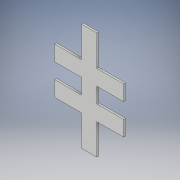
# Autodesk Inventor part: backplatelift
Saved by Autodesk Inventor 2017 (Build 210142000, 142)
## iProperties
Created: 2017-05-30
Part Number: backplatelift
Material: Generic
Document SubType Name: Modeling
Designer: User
Density: 1 g/cm^3
Appearance: Default
Author: User
Autodesk Inventor part; units mm, degrees
ref_plane "YZ Plane" through (0, 0, 0) normal (1, 0, 0) x (0, 1, 0)
ref_plane "XZ Plane" through (0, 0, 0) normal (0, 1, 0) x (-1, 0, 0)
ref_plane "XY Plane" through (0, 0, 0) normal (0, 0, 1) x (1, 0, 0)
sketch "Sketch1" plane through (0, 0, 0) normal (0, 0, 1) x (1, 0, 0)
  line L0 (0, 0) -> (50.8, 0)
  line L1 (50.8, 0) -> (50.8, 355.6)
  line L2 (50.8, 355.6) -> (0, 355.6)
  line L3 (0, 355.6) -> (0, 0)
  dimension "d0" = 50.8
  dimension "d1" = 355.6
  constraints: 8 end point, 2 parallel, 1 horizontal, 1 perpendicular
  measures "d0" distance of L2.end L1.end
  measures "d1" distance of L1.end L0.end
extrude "Extrusion1" add sketch "Sketch1" along normal blind 6.35
sketch "Sketch2" plane through (0, 0, 6.35) normal (0, 0, 1) x (1, 0, 0)
  line L0 (50.8, 0) -> (50.8, 355.6) projected
  line L1 (50.8, 152.4) -> (50.8, 203.2)
  line L2 (0, 152.4) -> (0, 203.2)
  line L3 (0, 355.6) -> (0, 0) projected
  line L4 (-88.9, 254) -> (0, 254)
  line L5 (0, 254) -> (0, 203.2)
  line L6 (0, 203.2) -> (-88.9, 203.2)
  line L7 (-88.9, 203.2) -> (-88.9, 254)
  line L8 (-88.9, 152.4) -> (0, 152.4)
  line L9 (0, 152.4) -> (0, 101.6)
  line L10 (0, 101.6) -> (-88.9, 101.6)
  line L11 (-88.9, 101.6) -> (-88.9, 152.4)
  line L12 (50.8, 101.6) -> (139.7, 101.6)
  line L13 (139.7, 101.6) -> (139.7, 152.4)
  line L14 (139.7, 152.4) -> (50.8, 152.4)
  line L15 (50.8, 152.4) -> (50.8, 101.6)
  line L16 (139.7, 203.2) -> (50.8, 203.2)
  line L17 (50.8, 203.2) -> (50.8, 254)
  line L18 (50.8, 254) -> (139.7, 254)
  line L19 (139.7, 254) -> (139.7, 203.2)
  point P0 (50.8, 152.4)
  point P1 (-88.9, 107.5788)
  point P2 (0, 254)
  constraints: 36 end point, 8 parallel, 5 point on line, 4 horizontal, 4 perpendicular
extrude "Extrusion3" add sketch "Sketch2" against normal blind 6.35
body "Solid1"
